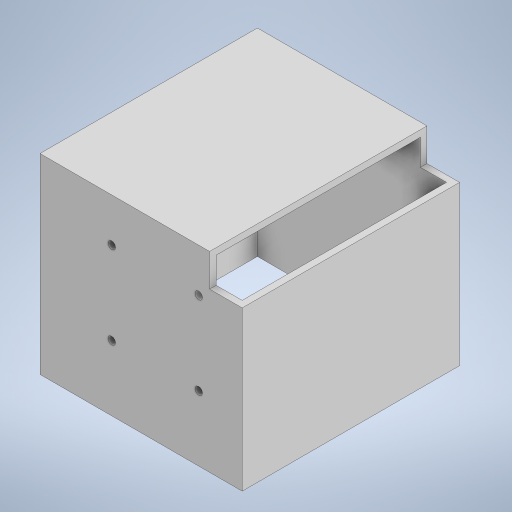
# Autodesk Inventor part: support_imu
Saved by Autodesk Inventor 2024 (Build 280153000, 153)
## iProperties
Created: 2023-10-03
Part Number: support_imu
Material: Générique
Document SubType Name: Modeling
Designer: apolline
Density: 1 g/cm^3
Appearance: Par défaut
Author: apolline
## iProperties of the stored document support_imu_Impression 3D.ipt
Created: 2023-10-03
Part Number: support_imu_Impression 3D
Material: Générique
Document SubType Name: Modeling
Designer: apolline
Density: 1 g/cm^3
Appearance: Par défaut
Author: apolline
Autodesk Inventor part; units mm, degrees
ref_plane "YZ Plane" through (0, 0, 0) normal (1, 0, 0) x (0, 1, 0)
ref_plane "XZ Plane" through (0, 0, 0) normal (0, 1, 0) x (-1, 0, 0)
ref_plane "XY Plane" through (0, 0, 0) normal (0, 0, 1) x (1, 0, 0)
sketch "Esquisse1" plane through (0, 0, 0) normal (0, 1, 0) x (-1, 0, 0)
  line L0 (-46.5, 50) -> (46.5, 50)
  line L1 (46.5, 50) -> (46.5, -50)
  line L2 (46.5, -50) -> (-46.5, -50)
  line L3 (-46.5, -50) -> (-46.5, 50)
  line L4 (-46.5, 50) -> (46.5, -50) construction
  line L5 (46.5, 50) -> (-46.5, -50) construction
  point P0 (0, 0)
  dimension "d0" = 100
  dimension "d1" = 93
  constraints: 12 end point, 2 midpoint, 2 parallel, 1 horizontal, 1 perpendicular
  measures "d0" distance of L0.end L1.end
  measures "d1" distance of L1.end L2.end
extrude "Extrusion1" add sketch "Esquisse1" along normal blind 88
sketch "Esquisse2" plane through (0, 0, 0) normal (0, -1, 0) x (1, 0, 0)
  line L0 (-43.5, 47) -> (43.5, 47)
  line L1 (43.5, 47) -> (43.5, -47)
  line L2 (43.5, -47) -> (-43.5, -47)
  line L3 (-43.5, -47) -> (-43.5, 47)
  line L4 (-43.5, 47) -> (43.5, -47) construction
  line L5 (43.5, 47) -> (-43.5, -47) construction
  line L6 (46.5, 50) -> (46.5, -50) projected
  line L7 (-46.5, 50) -> (46.5, 50) projected
  point P0 (0, 0)
  dimension "d4" = 3
  dimension "d5" = 3
  constraints: 12 end point, 2 midpoint, 2 parallel, 1 horizontal, 1 perpendicular
  measures "d4" distance between parallel lines of L6 L1
  measures "d5" distance between parallel lines of L7 L0
extrude "Extrusion2" cut sketch "Esquisse2" against normal blind 85
sketch "Esquisse3" plane through (-46.5, 0, 50) normal (0, 0, 1) x (1, 0, 0)
  line L0 (0, 88) -> (93, 88) projected
  line L1 (93, 88) -> (78, 88)
  line L2 (78, 88) -> (78, 73)
  line L3 (78, 73) -> (93, 73)
  line L4 (93, 73) -> (93, 88)
  point P0 (46.5, 0)
  dimension "d8" = 15
  dimension "d9" = 15
  constraints: 8 end point, 2 parallel, 1 horizontal, 1 perpendicular
  measures "d8" distance of L2.end L3.end
  measures "d9" distance of L1.end L2.end
extrude "Extrusion3" cut sketch "Esquisse3" against normal up to surface (100 mm away)
sketch "Esquisse4" plane through (-46.5, 0, 50) normal (0, 0, 1) x (1, 0, 0)
  circle A0 centre (73, 68) radius 1.75
  circle A1 centre (33, 68) radius 1.75
  circle A2 centre (73, 30) radius 1.75
  circle A3 centre (33, 30) radius 1.75
  line L0 (93, 0) -> (93, 73) projected
  line L1 (0, 88) -> (78, 88) projected
  point P0 (46.5, 0)
  dimension "d12" = 40
  dimension "d13" = 3.5
  dimension "d14" = 3.5
  dimension "d15" = 3.5
  dimension "d16" = 3.5
  dimension "d17" = 40
  dimension "d18" = 0
  dimension "d19" = 0
  dimension "d20" = 38
  dimension "d21" = 20
  dimension "d22" = 20
  dimension "d23" = 0
  constraints: 4 centre point
  measures "d12" distance of A0.centre A1.centre
  measures "d13" diameter of A1
  measures "d14" diameter of A0
  measures "d15" diameter of A2
  measures "d16" diameter of A3
  measures "d17" distance of A2.centre A3.centre
  measures "d18" vertical distance of A2.centre A3.centre
  measures "d19" horizontal distance of A0.centre A2.centre
  measures "d20" distance of A0.centre A2.centre
  measures "d21" distance from line of L0 A0.centre
  measures "d22" distance from line of L1 A0.centre
  measures "d23" vertical distance of A0.centre A1.centre
extrude "Extrusion4" cut sketch "Esquisse4" against normal up to surface (3 mm away)
sketch "Esquisse5" plane through (46.5, 0, -50) normal (0, 0, -1) x (-1, 0, 0)
  circle A0 centre (66.8, 77) radius 2.1
  circle A1 centre (41.4, 77) radius 2.1
  circle A2 centre (11, 44.9) radius 2.1
  circle A3 centre (11, 7.4) radius 2.1
  line L0 (0, 0) -> (0, 73) projected
  line L1 (15, 88) -> (93, 88) projected
  line L2 (15, 88) -> (15, 73) projected
  line L3 (15, 73) -> (0, 73) projected
  circle A4 centre (83, 7.4) radius 2.1
  line L4 (93, 0) -> (93, 88) projected
  point P0 (46.5, 0)
  dimension "d26" = 4.2
  dimension "d27" = 4.2
  dimension "d28" = 4.2
  dimension "d29" = 4.2
  dimension "d30" = 11
  dimension "d31" = 0
  dimension "d32" = 11
  dimension "d33" = 0
  dimension "d34" = 37.5
  dimension "d35" = 25.4
  dimension "d36" = 26.4
  dimension "d37" = 28.1
  dimension "d38" = 4.2
  dimension "d39" = 0
  dimension "d40" = 10
  constraints: 5 centre point
  measures "d26" diameter of A3
  measures "d27" diameter of A2
  measures "d28" diameter of A1
  measures "d29" diameter of A0
  measures "d30" distance from line of L0 A3.centre
  measures "d31" horizontal distance of A3.centre A2.centre
  measures "d32" distance from line of L1 A1.centre
  measures "d33" vertical distance of A1.centre A0.centre
  measures "d34" distance of A3.centre A2.centre
  measures "d35" distance of A0.centre A1.centre
  measures "d36" distance from line of L2 A1.centre
  measures "d37" distance from line of L3 A2.centre
  measures "d38" diameter of A4
  measures "d39" vertical distance of A3.centre A4.centre
  measures "d40" distance from line of L4 A4.centre
extrude "Extrusion5" add sketch "Esquisse5" along normal blind 5.7
sketch "Esquisse6" plane through (-36.5, 7.4, -55.7) normal (0, 0, -1) x (-1, 0, 0)
  point P0 (-36.5, -7.4)
